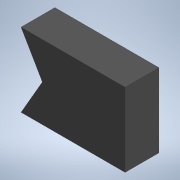
# Autodesk Inventor part: encajeTuerca
Saved by Autodesk Inventor 2021.5 (Build 255421000, 421)
## iProperties
Created: 2024-12-01
Part Number: encajeTuerca
Material: ABS NEGRO 4DLAB
Document SubType Name: Modeling
Designer: Joho_
Density: 1.075 g/cm^3
Appearance: Genérico(2)
Mass: 0.134706 g
Surface Area: 1.73218 cm^2
Volume: 0.125308 cm^3
Author: Joho_
## iProperties of the stored document _3DPrint.ipt
Created: 2024-12-01
Part Number: _3DPrint
Material: Genérico
Document SubType Name: Modeling
Designer: Joho_
Density: 1 g/cm^3
Appearance: Valor por defecto
Author: Joho_
Autodesk Inventor part; units mm, degrees
ref_plane "YZ Plane" through (0, 0, 0) normal (1, 0, 0) x (0, 1, 0)
ref_plane "XZ Plane" through (0, 0, 0) normal (0, 1, 0) x (-1, 0, 0)
ref_plane "XY Plane" through (0, 0, 0) normal (0, 0, 1) x (1, 0, 0)
sketch "Boceto1" plane through (0, 0, 0) normal (0, 0, 1) x (1, 0, 0)
  line L0 (15, 15) -> (15, 35)
  arc A0 (15, 2.5) -> (8.0075, 4.6388) centre (15, 15) ccw
  line L1 (15, -5) -> (18.5355, -1.4645) construction
  circle A1 centre (24.9038, 5.0962) radius 1.5
  line L2 (15, 15) -> (21.2936, 15)
  line L3 (30, 30) -> (0, 30)
  line L4 (0, 30) -> (0, 0)
  line L5 (0, 0) -> (30, 0)
  line L6 (30, 0) -> (30, 30)
  line L7 (30, 30) -> (0, 0) construction
  line L8 (23.3161, 2.3462) -> (21.7284, 5.0962)
  line L9 (21.7284, 5.0962) -> (23.3161, 7.8462)
  line L10 (23.3161, 7.8462) -> (26.4915, 7.8462)
  line L11 (26.4915, 7.8462) -> (28.0792, 5.0962)
  line L12 (28.0792, 5.0962) -> (26.4915, 2.3462)
  line L13 (26.4915, 2.3462) -> (23.3161, 2.3462)
  line L14 (28.0792, 24.9038) -> (26.4915, 27.6538)
  line L15 (23.3161, 22.1538) -> (26.4915, 22.1538)
  line L16 (21.7284, 24.9038) -> (23.3161, 22.1538)
  line L17 (26.4915, 22.1538) -> (28.0792, 24.9038)
  circle A2 centre (24.9038, 24.9038) radius 1.5
  line L18 (23.3161, 27.6538) -> (21.7284, 24.9038)
  line L19 (26.4915, 27.6538) -> (23.3161, 27.6538)
  line L20 (6.6839, 7.8462) -> (3.5085, 7.8462)
  line L21 (1.9208, 5.0962) -> (3.5085, 2.3462)
  line L22 (6.6839, 2.3462) -> (8.2716, 5.0962)
  circle A3 centre (5.0962, 5.0962) radius 1.5
  line L23 (8.2716, 5.0962) -> (6.6839, 7.8462)
  line L24 (8.2716, 24.9038) -> (6.6839, 22.1538)
  line L25 (6.6839, 22.1538) -> (3.5085, 22.1538)
  line L26 (3.5085, 22.1538) -> (1.9208, 24.9038)
  line L27 (1.9208, 24.9038) -> (3.5085, 27.6538)
  line L28 (6.6839, 27.6538) -> (8.2716, 24.9038)
  line L29 (3.5085, 27.6538) -> (6.6839, 27.6538)
  line L30 (3.5085, 7.8462) -> (1.9208, 5.0962)
  circle A4 centre (5.0962, 24.9038) radius 1.5
  line L31 (3.5085, 2.3462) -> (6.6839, 2.3462)
  line L32 (6.8282, 27.9038) -> (8.5603, 24.9038)
  line L33 (8.5603, 24.9038) -> (6.8282, 21.9038)
  line L34 (6.8282, 21.9038) -> (3.3641, 21.9038)
  line L35 (3.3641, 21.9038) -> (1.6321, 24.9038)
  line L36 (1.6321, 24.9038) -> (3.3641, 27.9038)
  line L37 (3.3641, 27.9038) -> (6.8282, 27.9038)
  line L38 (3.3641, 8.0962) -> (6.8282, 8.0962)
  line L39 (8.416, 4.8462) -> (8.2165, 4.5007)
  line L40 (6.8282, 2.0962) -> (3.3641, 2.0962)
  line L41 (3.3641, 2.0962) -> (1.6321, 5.0962)
  line L42 (1.6321, 5.0962) -> (3.3641, 8.0962)
  line L43 (15, 22.8053) -> (15, 21.1553)
  line L44 (6.8282, 27.9038) -> (15, 27.9038)
  line L45 (15, 27.9038) -> (15, 21.9038)
  line L46 (15, 21.9038) -> (6.8282, 21.9038)
  line L47 (6.8282, 21.9038) -> (6.8282, 27.9038)
  line L48 (6.8282, 2.0962) -> (15, 2.0962)
  line L49 (15, 2.0962) -> (15, 8.0962)
  line L50 (15, 8.0962) -> (6.8282, 8.0962)
  line L51 (6.8282, 7.5962) -> (6.8282, 2.5962)
  line L52 (8.416, 5.3462) -> (8.5603, 5.0962)
  line L53 (6.5396, 2.0962) -> (8.2716, 5.0962)
  line L54 (8.416, 5.3462) -> (8.7064, 5.8492)
  line L55 (6.5396, 8.0962) -> (8.2716, 5.0962)
  line L56 (8.416, 4.8462) -> (8.5603, 4.5962)
  point P0 (0, 0)
  point P1 (30, 5)
  point P2 (15, 15)
  point P3 (24.9038, 24.9038)
  point P4 (8.7064, 15)
  point P5 (15, 22.3631)
  point P6 (6.8282, 8.0962)
  point P7 (6.8282, 21.9038)
  point P8 (15, 21.9038)
  point P9 (15, 27.9038)
  point P10 (8.2716, 5.0962)
  dimension "d0" = 25
  dimension "d1" = 3
  dimension "d2" = 30
  dimension "d3" = 30
  dimension "d4" = 0.25
  dimension "d5" = 0.25
  constraints: 114 end point, 9 point on line, 5 centre point, 4 parallel, 2 horizontal, 2 perpendicular, 2 point on circle, 1 midpoint, 20 other
  measures "d0" diameter of A0
  measures "d1" diameter of A1
  measures "d2" distance of L5.end L4.end
  measures "d3" distance of L4.end L3.end
  measures "d4" distance between parallel lines of L29 L37
  measures "d5" distance between parallel lines of L20 L38
extrude "Extrusión1" add sketch "Boceto1" along normal blind 2.75 contours L38 L50 L49 L48 L40 L53 L22 L23 L55
